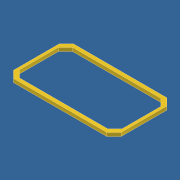
# Autodesk Inventor part: клей
Saved by Autodesk Inventor 2012 (Build 160160000, 160)
## iProperties
Created: 2009-09-08
Part Number: клей
Material: По умолчанию
Document SubType Name: Обычные детали
Designer: toma
Density: 1 g/cm^3
Mass: 0.668 g
Surface Area: 13.6251 cm^2
Volume: 0.668 cm^3
Sheet Metal Rule: По умолчанию_мм
Author: toma
Autodesk Inventor part; units mm, degrees
ref_plane "YZ Plane" through (0, 0, 0) normal (1, 0, 0) x (0, 1, 0)
ref_plane "XZ Plane" through (0, 0, 0) normal (0, 1, 0) x (-1, 0, 0)
ref_plane "XY Plane" through (0, 0, 0) normal (0, 0, 1) x (1, 0, 0)
sketch "Эскиз1" plane through (0, 0, 0) normal (0, 0, 1) x (1, 0, 0)
  line L0 (-16, -10) -> (34, -10)
  line L1 (38, -6) -> (38, 16)
  line L2 (34, 20) -> (-16, 20)
  line L3 (-20, 16) -> (-20, -6)
  line L4 (-20, 16) -> (-16, 20)
  line L5 (-16, -10) -> (-20, -6)
  line L6 (34, 20) -> (38, 16)
  line L7 (34, -10) -> (38, -6)
  line L8 (-18, -13.8) -> (-18, 33.1) construction
  line L9 (36, -15.5) -> (36, 27.4) construction
  line L10 (-22.5, 15) -> (39.4, 15) construction
  line L11 (-26.6, 10) -> (40.2, 10) construction
  line L12 (-27.2, 5) -> (41.5, 5) construction
  line L13 (-27.8, 0) -> (41.6, 0) construction
  line L14 (-27.6, -5) -> (40.5, -5) construction
  line L15 (-17.5, -12) -> (35.5, -12)
  line L16 (39.5, -8) -> (39.5, 18)
  line L17 (35.5, 22) -> (-17.5, 22)
  line L18 (-21.5, 18) -> (-21.5, -8)
  line L19 (-21.5, 18) -> (-17.5, 22)
  line L20 (39.5, -8) -> (35.5, -12)
  line L21 (39.5, 18) -> (35.5, 22)
  line L22 (39.5, -8) -> (35.5, -12)
  line L23 (-21.5, -8) -> (-17.5, -12)
  point P0 (-20, -10)
  point P1 (38, 20)
  point P2 (38, -10)
  point P3 (-20, 20)
  point P4 (-18, 15)
  point P5 (-18, 10)
  point P6 (-18, 5)
  point P7 (36, 15)
  point P8 (36, 10)
  point P9 (36, 5)
  point P10 (36, 0)
  point P11 (36, -5)
  point P12 (-21.5, -12)
  point P13 (39.5, 22)
  point P14 (39.5, -12)
  point P15 (-21.5, 22)
  point P16 (39.5, -12)
  dimension "d0" = 58
  dimension "d1" = 30
  dimension "d2" = 4
  dimension "d3" = 4
  dimension "d4" = 4
  dimension "d5" = 4
  dimension "d6" = 4
  dimension "d7" = 4
  dimension "d8" = 4
  dimension "d9" = 4
  dimension "d12" = 2
  dimension "d13" = 2
  dimension "d14" = 5
  dimension "d15" = 5
  dimension "d16" = 5
  dimension "d17" = 5
  dimension "d18" = 5
  dimension "d42" = 2
  dimension "d43" = 2
  dimension "d44" = 1.5
  dimension "d45" = 1.5
  dimension "d46" = 4
  dimension "d47" = 4
  dimension "d48" = 4
  dimension "d49" = 4
  dimension "d50" = 4
  dimension "d51" = 4
  dimension "d52" = 4
  dimension "d53" = 4
  dimension "d54" = 4
  dimension "d55" = 4
  constraints: 48 end point, 36 point on line, 9 parallel, 3 perpendicular, 2 horizontal
  measures "d0" distance of point (38, 20) point (-20, 20)
  measures "d1" distance of point (-20, 20) point (-20, -10)
  measures "d2" distance of L3.start point (-20, 20)
  measures "d3" distance of L2.end point (-20, 20)
  measures "d4" distance of L0.start point (-20, -10)
  measures "d5" distance of L3.end point (-20, -10)
  measures "d6" distance of L2.start point (38, 20)
  measures "d7" distance of L1.end point (38, 20)
  measures "d8" distance of L0.end point (38, -10)
  measures "d9" distance of L1.start point (38, -10)
  measures "d12" distance between parallel lines of L8 L3
  measures "d13" distance between parallel lines of L9 L1
  measures "d14" distance between parallel lines of L10 L2
  measures "d15" distance between parallel lines of L11 L10
  measures "d16" distance between parallel lines of L12 L11
  measures "d17" distance between parallel lines of L13 L12
  measures "d18" distance between parallel lines of L13 L14
  measures "d42" distance between parallel lines of L17 L2
  measures "d43" distance between parallel lines of L0 L15
  measures "d44" distance between parallel lines of L18 L3
  measures "d45" distance between parallel lines of L1 L16
  measures "d46" distance of L18.start point (-21.5, 22)
  measures "d47" distance of L17.end point (-21.5, 22)
  measures "d48" distance of L20.start point (39.5, -12)
  measures "d49" distance of L20.end point (39.5, -12)
  measures "d50" distance of L16.end point (39.5, 22)
  measures "d51" distance of L17.start point (39.5, 22)
  measures "d52" distance of L16.start point (39.5, -12)
  measures "d53" distance of L15.end point (39.5, -12)
  measures "d54" distance of L18.end point (-21.5, -12)
  measures "d55" distance of L15.start point (-21.5, -12)
extrude "Выдавливание2" add sketch "Эскиз1" along normal blind 2
equation "\"d3\" = d2"
equation "\"d4\" = d2"
equation "\"d5\" = d4"
equation "\"d6\" = d2"
equation "\"d7\" = d6"
equation "\"d8\" = d2"
equation "\"d9\" = d8"
equation "\"d47\" = d46"
equation "\"d49\" = d48"
equation "\"d51\" = d50"
equation "\"d53\" = d52"
equation "\"d54\" = d52"
equation "\"d55\" = d54"
equation "\"Радиус_гибки\" = Толщина"
equation "\"Ширина_просечки\" = Толщина"
equation "\"Глубина_просечки\" = 0.5 * Толщина"
equation "\"Размер_высечки\" = 4 * Толщина"
equation "\"Мин_остаток\" = 2 * Толщина"
equation "\"Радиус_перехода\" = Радиус_гибки"
equation "\"Радиус_Якоби\" = Радиус_гибки"
equation "\"Размер_зазора\" = Толщина"
equation "\"Толщина\" = 0.5"
